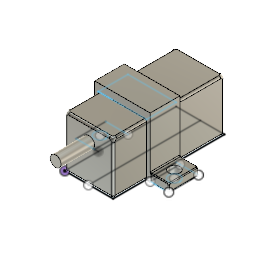
Maze Solver (Autodesk Fusion 360 archive; units mm, degrees)
design "Motor"
part number: 2025-08-21-21-51-39-683
Autodesk Fusion 360 part; units mm, degrees
note: some values were not read from the file. Chosen so that the rebuilt part matches the saved one: which face or edge a step refers to; which pieces of a blend or face edit are solid. Set by a fixed rule: which sketch regions a step uses.
sketch "Sketch1" plane through (0, 0, 0) normal (0, 0, 1) x (1, 0, 0)
  line L0 (0, 0) -> (13, 0)
  line L1 (13, 0) -> (13, 30)
  line L2 (13, 30) -> (0, 30)
  line L3 (0, 30) -> (0, 0)
  line L4 (13, 17.0121) -> (14, 17.0121)
  line L5 (14, 17.0121) -> (14, 9)
  line L6 (14, 9) -> (13, 9)
  line L7 (13, 9) -> (13, 17.0121)
  line L8 (6.5, 30) -> (6.5, -0.1417)
  line L9 (0, 17.0121) -> (-1, 17.0121)
  line L10 (-1, 9) -> (0, 9)
  line L11 (-1, 9.0098) -> (-6, 9.0098)
  line L12 (-6, 9.0098) -> (-6, 17.0098)
  line L13 (-6, 17.0098) -> (-1, 17.0098)
  line L14 (-1, 17.0098) -> (-1, 9.0098)
  circle A0 centre (-3.5, 13) radius 1.5
  circle A1 centre (16.5, 13) radius 1.5
  line L15 (19, 9.0098) -> (19, 17.0098)
  line L16 (19, 17.0098) -> (14, 17.0098)
  line L17 (14, 9.0098) -> (19, 9.0098)
  line L18 (-1, 17.0121) -> (-1, 17.0098)
  line L19 (-1, 9.0098) -> (-1, 9)
  dimension "d5" = 30
  dimension "d8" = 8
  dimension "d10" = 3
  dimension "d12" = 10
  dimension "d13" = 13
  dimension "d16" = 1
  dimension "d17" = 5
  dimension "d24" = 9
  constraint horizontal L0
  constraint vertical L1
  constraint horizontal L2
  constraint vertical L3
  constraint coincident L0.start L3.end
  constraint horizontal L4
  constraint vertical L5
  constraint horizontal L6
  constraint vertical L7
  constraint coincident L1 L4.start
  constraint midpoint L2 L8.start
  constraint perpendicular L0 L8
  constraint symmetric L4.start L8 L9.start
  constraint symmetric L4.end L8 L9.end
  constraint symmetric L5.end L8 L10.start
  constraint symmetric L6.end L8 L10.end
  constraint horizontal L11
  constraint vertical L12
  constraint horizontal L13
  constraint vertical L14
  constraint coincident L11.start L18
  constraint symmetric L8 L11.end L15.start
  constraint symmetric L8 L12.end L15.end
  constraint symmetric L8 A0 A1
  constraint symmetric L8 L11.start L17.start
  constraint symmetric L8 L13.end L16.end
  constraint collinear L18 L19
  measures "d5" distance of L0.start L2.end
  measures "d8" distance of L11.start L13.end
  measures "d10" diameter of A0
  measures "d12" distance of L8 A0.centre
  measures "d13" distance of L0.start L0.end
  measures "d16" distance of L9.end L9.start
  measures "d17" distance of L11.start L11.end
  measures "d24" distance of L0.start L10.end
extrude "Extrude3" add sketch "Sketch1" along normal blind 2 contours L11 L12 L13 L14 | L5 L15 L16 L17 makes body 1 at (-3.4626, 16.1718, 0) makes body 2 at (16.5374, 16.1718, 0)
fillet "Fillet1" radius 0.2 10 edges at (-6, 9.0098, 1) (-3.5, 9.0098, 2) (-6, 17.0098, 1) (-6, 13.0098, 2) (-3.5, 17.0098, 2) (19, 17.0098, 1) (16.5, 17.0098, 2) (19, 9.0098, 1) (19, 13.0098, 2) (16.5, 9.0098, 2) on bodies 1 2
ref_plane "WorkPlane2" through (6.5, 0, 5) normal (0, -1, 0) x (1, 0, 0)
sketch "Sketch3" plane through (0, 0, 0) normal (0, -1, 0) x (-1, 0, 0)
  circle A0 centre (-6.5, -10) radius 1.5
  point P0 (-6.5, 0)
  dimension "d42" = 3
  dimension "d66" = 10
  measures "d42" diameter of A0
  measures "d66" distance of A0.centre P0
extrude "Extrude7" add sketch "Sketch1" along normal blind 14 separate body contours L0 L2 L3 L8 | L0 L1 L2 L7 L8 makes body 3
extrude "Extrude8" add sketch "Sketch1" along normal blind 16 contours L3 L9 L10 L14 L18 L19 | L1 L4 L5 L6 L7 bodies 1 2 3
ref_plane "WorkPlane3" through (6.5, 15, 14) normal (0, 0, 1) x (1, 0, 0)
sketch "Sketch5" plane through (0, 0, 14) normal (0, 0, 1) x (1, 0, 0)
  line L0 (0, 17) -> (13, 17)
  line L1 (13, 17) -> (13, 9)
  line L2 (13, 9) -> (0, 9)
  line L3 (0, 9) -> (0, 17)
  constraint horizontal L0
  constraint vertical L1
  constraint horizontal L2
  constraint vertical L3
extrude "Extrude9" add sketch "Sketch5" along normal blind 2 bodies 1
extrude "Extrude10" add sketch "Sketch3" along normal blind 9 bodies 1
fillet "Fillet5" radius 0.25 5 edges at (-1, 9.0098, 0.9) (-1, 9.0684, 1.9414) (-1, 13.0098, 2) (-1, 16.9512, 1.9414) (-1, 17.0098, 0.9) on bodies 1
fillet "Fillet6" radius 0.25 5 edges at (14, 17.0098, 0.9) (14, 16.9512, 1.9414) (14, 13.0098, 2) (14, 9.0684, 1.9414) (14, 9.0098, 0.9) on bodies 1
fillet "Fillet7" radius 0.5 10 edges at (0, 4.5, 14) (6.5, 0, 14) (13, 4.5, 14) (0, 0, 7) (13, 0, 7) (0, 30, 7) (0, 23.506, 14) (13, 23.506, 14) (6.5, 30, 14) (13, 30, 7) on bodies 1 3
fillet "Fillet8" radius 0.5 5 edges at (0, 4.75, 0) (0.1464, 0.1464, 0) (6.5, 0, 0) (12.8536, 0.1464, 0) (13, 4.75, 0) on bodies 1
fillet "Fillet9" radius 0.5 5 edges at (13, 23.256, 0) (12.8536, 29.8536, 0) (6.5, 30, 0) (0.1464, 29.8536, 0) (0, 23.256, 0) on bodies 1
extrude "Extrude6" [suppressed]
fillet "Fillet2" [suppressed]
